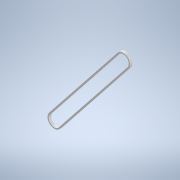
# Autodesk Inventor part: Lift down banding
Saved by Autodesk Inventor 2022.2 (Build 262287010, 287A)
## iProperties
Created: 2022-06-27
Part Number: Lift down banding
Material: Generic
Document SubType Name: Modeling
Designer: Main Account
Density: 1 g/cm^3
Appearance: Default
Author: Main Account
Autodesk Inventor part; units mm, degrees
ref_plane "YZ Plane" through (0, 0, 0) normal (1, 0, 0) x (0, 1, 0)
ref_plane "XZ Plane" through (0, 0, 0) normal (0, 1, 0) x (-1, 0, 0)
ref_plane "XY Plane" through (0, 0, 0) normal (0, 0, 1) x (1, 0, 0)
sketch "Sketch1" plane through (0, 0, 0) normal (0, 0, 1) x (1, 0, 0)
  arc A0 (-8.9464, 7.1138) -> (8.9464, -7.1138) centre (0, 0) ccw
  arc A1 (148.494, 168.382) -> (130.6012, 182.6097) centre (139.5476, 175.4959) ccw
  line L0 (-8.9464, 7.1138) -> (130.6012, 182.6097)
  line L1 (148.494, 168.382) -> (8.9464, -7.1138)
  arc A2 (-10.9345, 8.6947) -> (10.9345, -8.6947) centre (0, 0) ccw
  arc A3 (150.4821, 166.8012) -> (128.6131, 184.1906) centre (139.5476, 175.4959) ccw
  line L2 (128.6131, 184.1906) -> (-10.9345, 8.6947)
  line L3 (150.4821, 166.8012) -> (10.9345, -8.6947)
  dimension "d0" = 22.86
  dimension "d1" = 22.86
  dimension "d3" = 27.94
  dimension "d4" = 27.94
  constraints: 8 end point, 8 point on circle, 8 tangent, 4 centre point, 3 coincident
  measures "d0" diameter of A0
  measures "d1" diameter of A1
  measures "d3" diameter of A2
  measures "d4" diameter of A3
extrude "Extrusion1" add sketch "Sketch1" against normal blind 5.08
body "Solid1"
